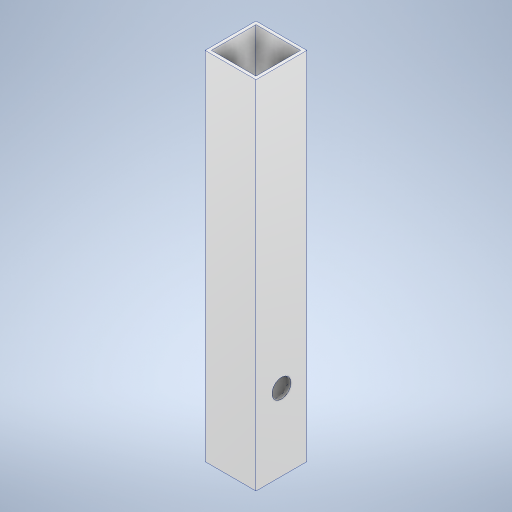
# Autodesk Inventor part: Tube Finger
Saved by Autodesk Inventor 2024 (Build 280153000, 153)
## iProperties
Created: 2023-09-27
Part Number: Tube Finger
Material: Aluminum 6061
Document SubType Name: Modeling
Designer: Megan
Density: 2.7 g/cm^3
Appearance: Aluminum - Flat
Author: Megan
Autodesk Inventor part; units mm, degrees
ref_plane "YZ Plane" through (0, 0, 0) normal (1, 0, 0) x (0, 1, 0)
ref_plane "XZ Plane" through (0, 0, 0) normal (0, 1, 0) x (-1, 0, 0)
ref_plane "XY Plane" through (0, 0, 0) normal (0, 0, 1) x (1, 0, 0)
sketch "Sketch1" plane through (0, 0, 0) normal (0, 1, 0) x (-1, 0, 0)
  line L0 (12.7, 12.7) -> (12.7, -12.7)
  line L1 (12.7, -12.7) -> (-12.7, -12.7)
  line L2 (-12.7, -12.7) -> (-12.7, 12.7)
  line L3 (-12.7, 12.7) -> (12.7, 12.7)
  line L4 (12.7, 12.7) -> (-12.7, -12.7) construction
  line L5 (12.7, -12.7) -> (-12.7, 12.7) construction
  line L6 (11.1125, 11.1125) -> (11.1125, -11.1125)
  line L7 (11.1125, -11.1125) -> (-11.1125, -11.1125)
  line L8 (-11.1125, -11.1125) -> (-11.1125, 11.1125)
  line L9 (-11.1125, 11.1125) -> (11.1125, 11.1125)
  line L10 (11.1125, 11.1125) -> (-11.1125, -11.1125) construction
  line L11 (11.1125, -11.1125) -> (-11.1125, 11.1125) construction
  point P0 (0, 0)
  dimension "d0" = 25.4
  dimension "d1" = 25.4
  dimension "d2" = 1.5875
  dimension "d3" = 1.5875
  constraints: 24 end point, 4 midpoint, 4 parallel, 2 perpendicular, 2 vertical
  measures "d0" distance of L0.start L0.end
  measures "d1" distance of L0.end L1.end
  measures "d2" distance between parallel lines of L0 L6
  measures "d3" distance between parallel lines of L1 L7
extrude "Extrusion1" add sketch "Sketch1" along normal blind 660.4
sketch "Sketch2" plane through (12.7, 0, 12.7) normal (1, 0, 0) x (0, 0, -1)
  line L0 (12.7, 0) -> (12.7, 38.1)
  circle A0 centre (12.7, 38.1) radius 4.7625
  line L1 (3.9688, 38.1) -> (8.3344, 45.6615)
  line L2 (8.3344, 45.6615) -> (17.0656, 45.6615)
  line L3 (17.0656, 45.6615) -> (21.4313, 38.1)
  line L4 (21.4313, 38.1) -> (17.0656, 30.5385)
  line L5 (17.0656, 30.5385) -> (8.3344, 30.5385)
  line L6 (8.3344, 30.5385) -> (3.9688, 38.1)
  dimension "d6" = 38.1
  dimension "d7" = 9.525
  dimension "d8" = 8.7312
  constraints: 14 end point, 2 coincident, 1 centre point, 1 vertical, 13 other
  measures "d6" distance of L0.start L0.end
  measures "d7" diameter of A0
  measures "d8" distance of L0.end L1.start
extrude "Extrusion2" cut sketch "Sketch2" against normal blind 46.6 contours A0
sketch "Sketch3" plane through (12.7, 0, 12.7) normal (1, 0, 0) x (0, 0, -1)
  line L0 (12.7, 0) -> (12.7, 177.8)
  line L1 (0, 0) -> (0, 660.4) projected
  line L2 (0, 177.8) -> (180.4268, 177.8)
  line L3 (180.4268, 177.8) -> (180.4268, 742.2297)
  line L4 (180.4268, 742.2297) -> (0, 742.2297)
  line L5 (0, 742.2297) -> (0, 177.8)
  dimension "d11" = 177.8
  constraints: 10 end point, 2 parallel, 1 horizontal, 1 perpendicular, 1 point on line, 1 vertical
  measures "d11" distance of L0.start L0.end
extrude "Extrusion3" cut sketch "Sketch3" against normal blind 354.85
body "Solid1"
